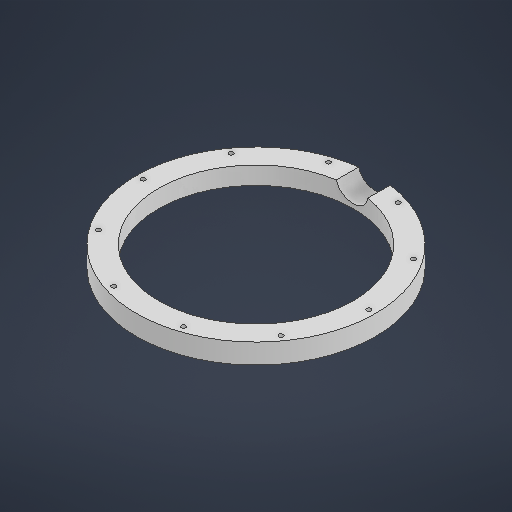
# Autodesk Inventor part: Cylinder Bottom
Saved by Autodesk Inventor 2025 (Build 290162000, 162)
## iProperties
Created: 2024-04-29
Part Number: Cylinder Bottom
Material: Generic
Document SubType Name: Modeling
Designer: Thienan Hoang
Density: 1 g/cm^3
Appearance: Default
Author: Thienan Hoang
Autodesk Inventor part; units mm, degrees
ref_plane "YZ Plane" through (0, 0, 0) normal (1, 0, 0) x (0, 1, 0)
ref_plane "XZ Plane" through (0, 0, 0) normal (0, 1, 0) x (-1, 0, 0)
ref_plane "XY Plane" through (0, 0, 0) normal (0, 0, 1) x (1, 0, 0)
sketch "Sketch1" plane through (0, 0, 0) normal (0, 1, 0) x (-1, 0, 0)
  circle A0 centre (0, 0) radius 135
  circle A1 centre (0, 0) radius 110
  dimension "d0" = 270
  dimension "d1" = 220
  constraints: 2 centre point, 2 coincident
  measures "d0" diameter of A0
  measures "d1" diameter of A1
extrude "Extrusion1" add sketch "Sketch1" along normal blind 20
sketch "Sketch2" plane through (0, 0, 0) normal (0, 0, 1) x (1, 0, 0)
  circle A0 centre (0, 23) radius 18
  line L0 (135, 0) -> (-135, 0) projected
  point P0 (0, 0)
  dimension "d4" = 36
  dimension "d5" = 23
  constraints: 1 centre point
  measures "d4" diameter of A0
  measures "d5" distance from line of L0 A0.centre
extrude "Extrusion2" cut sketch "Sketch2" against normal through all
sketch "Sketch3" plane through (0, 20, 0) normal (0, 1, 0) x (1, 0, 0)
  circle A0 centre (0, 0) radius 127.5
  circle A1 centre (-127.5, 0) radius 2
  circle A2 centre (-103.1497, -74.9426) radius 2
  circle A3 centre (-39.3997, -121.2597) radius 2
  circle A4 centre (39.3997, -121.2597) radius 2
  circle A5 centre (103.1497, -74.9426) radius 2
  circle A6 centre (127.5, 0) radius 2
  circle A7 centre (103.1497, 74.9426) radius 2
  circle A8 centre (39.3997, 121.2597) radius 2
  circle A9 centre (-39.3997, 121.2597) radius 2
  circle A10 centre (-103.1497, 74.9426) radius 2
  dimension "d8" = 255
  dimension "d9" = 4
  dimension "d12" = 360
  constraints: 10 centre point, 1 coincident, 1 horizontal alignment, 23 other
  measures "d9" diameter of A1
hole "Hole1" at (103.1497, 20, 74.9426) at (127.5, 20, 0) at (103.1497, 20, -74.9426) at (39.3997, 20, -121.2597) at (-39.3997, 20, -121.2597) at (-103.1497, 20, -74.9426) at (-127.5, 20, 0) at (-103.1497, 20, 74.9426) at (-39.3997, 20, 121.2597) at (39.3997, 20, 121.2597) direction (0, -1, 0) diameter 5 end through all
sketch "Sketch4" plane through (0, 0, 0) normal (0, -1, 0) x (1, 0, 0)
  circle A0 centre (0, 0) radius 131.5
  circle A1 centre (0, 0) radius 135
  dimension "d21" = 263
  constraints: 2 centre point, 2 coincident
  measures "d21" diameter of A0
extrude "Extrusion3" add sketch "Sketch4" along normal blind 2.5
body "Solid1"
